measurement_tape_clip (Autodesk Fusion 360 design; units mm, degrees)
Autodesk Fusion 360 part; units mm, degrees
sketch "Sketch1" plane through (0, 0, 0) normal (0, 0, 1) x (1, 0, 0)
  circle A0 centre (0, 0) radius 13.5
  circle A1 centre (0, 0) radius 15.5
  line L0 (0, 0) -> (-5.3013, 14.5652)
  line L1 (0, 0) -> (5.3013, 14.5652)
  line L2 (0, 0) -> (0, 25)
  dimension "d1" = 27
  dimension "d2" = 31
  dimension "d3" = 20
  dimension "d4" = 20
  constraint coincident A0.centre A1.centre
  constraint concentric A0 A1
  constraint coincident A1 L0.end
  constraint coincident A1 L1.end
  constraint vertical L2
  measures "d1" diameter of A0
  measures "d2" diameter of A1
  measures "d3" angle of L1 L2
  measures "d4" angle of L0 L2
extrude "Extrude1" add sketch "Sketch1" along normal blind 12 contours A0 A1 L0 L1
fillet "Fillet1" radius 1 4 edges at (-5.3013, 14.5652, 6) (-4.6173, 12.6859, 6) (4.6173, 12.6859, 6) (5.3013, 14.5652, 6)
equation "d2 = d1 + 4 mm"
equation "d4 = d3"
